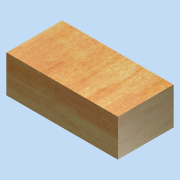
# Autodesk Inventor part: FrameBlock
Saved by Autodesk Inventor 2014 (Build 180170000, 170)
## iProperties
Created: 2012-05-22
Part Number: FrameBlock
Material: Generic
Document SubType Name: Modeling
Designer: dgitz
Density: 1 g/cm^3
Appearance: Yellow Pine - Solid Stained Light Low Gloss
d0: 1.500 in
d1: 0.500 in
d2: 0.750 in
d3: 0.00 deg
Author: dgitz
Autodesk Inventor part; units mm, degrees
ref_plane "YZ Plane" through (0, 0, 0) normal (1, 0, 0) x (0, 1, 0)
ref_plane "XZ Plane" through (0, 0, 0) normal (0, 1, 0) x (-1, 0, 0)
ref_plane "XY Plane" through (0, 0, 0) normal (0, 0, 1) x (1, 0, 0)
sketch "Sketch1" plane through (0, 0, 0) normal (0, 0, 1) x (1, 0, 0)
  line L0 (-19.05, 6.35) -> (19.05, 6.35)
  line L1 (19.05, 6.35) -> (19.05, -6.35)
  line L2 (19.05, -6.35) -> (-19.05, -6.35)
  line L3 (-19.05, -6.35) -> (-19.05, 6.35)
  line L4 (-19.05, -6.35) -> (19.05, 6.35) construction
  point P0 (0, 0)
  point P1 (0, 0)
  dimension "d0" = 38.1
  dimension "d1" = 12.7
  constraints: 10 end point, 2 parallel, 1 coincident, 1 horizontal, 1 midpoint, 1 perpendicular
  measures "d0" distance between parallel lines of L1 L3
  measures "d1" distance of L2.end L0.start
extrude "Extrusion1" add sketch "Sketch1" along normal mid plane 19.05
body "Solid1"
